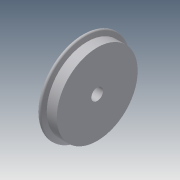
# Autodesk Inventor part: sprocket
Saved by Autodesk Inventor 2014 (Build 180170000, 170)
## iProperties
Created: 2016-01-12
Part Number: sprocket
Material: Generic
Document SubType Name: Modeling
Designer: Paul
Density: 1 g/cm^3
Appearance: Default
Author: Paul
Autodesk Inventor part; units mm, degrees
ref_plane "YZ Plane" through (0, 0, 0) normal (1, 0, 0) x (0, 1, 0)
ref_plane "XZ Plane" through (0, 0, 0) normal (0, 1, 0) x (-1, 0, 0)
ref_plane "XY Plane" through (0, 0, 0) normal (0, 0, 1) x (1, 0, 0)
sketch "Sketch1" plane through (0, 0, 0) normal (0, 0, 1) x (1, 0, 0)
  line L0 (3.556, 0) -> (10.414, 0)
  line L1 (3.556, 0) -> (3.556, 25.4)
  line L2 (3.556, 25.4) -> (0, 25.4)
  line L3 (0, 25.4) -> (0, 31.5852)
  line L4 (0, 31.5852) -> (-1.191, 34.8015)
  arc A0 (1.191, 35.6835) -> (-1.191, 34.8015) centre (0, 35.2425) ccw
  line L5 (1.191, 35.6835) -> (2.3183, 32.639)
  line L6 (2.3183, 32.639) -> (10.414, 32.639)
  line L7 (10.414, 32.639) -> (10.414, -88.0052)
  point P0 (0, 0)
  dimension "d0" = 25.4
  dimension "d1" = 36.5125
  dimension "d2" = 1.27
  dimension "d3" = 11.684
  dimension "d4" = 32.639
  dimension "d5" = 3.556
  constraints: 16 end point, 3 parallel, 3 perpendicular, 2 point on circle, 2 tangent, 2 vertical alignment, 1 centre point, 1 horizontal, 1 horizontal alignment, 1 point on line
  measures "d0" distance between parallel lines of L2 L0
  measures "d2" radius of A0
  measures "d4" distance between parallel lines of L6 L0
  measures "d5" distance between parallel lines of L1 L3
revolve "Revolution1" add sketch "Sketch1" angle 360 about axis through (3.556, 0, 0) along (1, 0, 0)
sketch "Sketch2" plane through (10.414, 0, 0) normal (1, 0, 0) x (0, 0, -1)
  circle A0 centre (0, 0) radius 32.639 projected
  circle A1 centre (0, 0) radius 4.7625
  dimension "d7" = 9.525
  constraints: 1 centre point, 1 coincident
  measures "d7" diameter of A1
extrude "Extrusion1" cut sketch "Sketch2" against normal blind 25.4 contours A1
body "Solid1"
